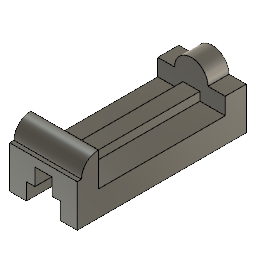
Task1 3C 2 v1 (Autodesk Fusion 360 design; units mm, degrees)
Autodesk Fusion 360 part; units mm, degrees
note: some values were not read from the file. Set by a fixed rule: which sketch regions a step uses.
sketch "Sketch1" plane through (0, 0, 0) normal (0, 0, 1) x (1, 0, 0) in component "box"
  line L0 (40, 100) -> (-40, 100)
  line L1 (-40, 100) -> (-40, -100)
  line L2 (-40, -100) -> (40, -100)
  line L3 (40, -100) -> (40, 100)
  line L4 (40, 100) -> (-40, -100) construction
  line L5 (-40, 100) -> (40, -100) construction
  dimension "d1" = 80
  dimension "d2" = 200
  constraint horizontal L0
  constraint perpendicular L0 L1
  constraint parallel L0 L2
  constraint parallel L1 L3
  constraint coincident L4 origin
  constraint coincident L5 origin
  measures "d1" distance of L1.end L2.end
  measures "d2" distance of L0.end L1.end
extrude "Extrude1" add sketch "Sketch1" along normal blind 50 in component "box"
sketch "Sketch2" plane through (0, -100, 0) normal (0, -1, 0) x (1, 0, 0) in component "box"
  line L0 (-40, 0) -> (40, 0)
  line L1 (40, 0) -> (40, 50)
  line L2 (40, 50) -> (-40, 50)
  line L3 (-40, 50) -> (-40, 0)
  line L4 (20, 0) -> (-20, 0)
  line L5 (-20, 0) -> (-20, 20)
  line L6 (-20, 20) -> (20, 20)
  line L7 (20, 20) -> (20, 0)
  line L8 (20, 0) -> (-20, 20) construction
  line L9 (-20, 0) -> (20, 20) construction
  point P0 (0, 10)
  constraint horizontal L4
  constraint perpendicular L4 L5
  constraint parallel L4 L6
  constraint parallel L5 L7
  constraint coincident L8 P0
  constraint coincident L9 P0
  constraint coincident L0 L4.start
extrude "Extrude2" cut sketch "Sketch2" against normal blind 200 contours L0 L4 L5 L6 L7 in component "box"
sketch "Sketch3" plane through (0, -100, 0) normal (0, -1, 0) x (1, 0, 0) in component "box"
  line L0 (20, 20) -> (20, 0)
  line L1 (20, 0) -> (40, 0)
  line L2 (40, 0) -> (40, 50)
  line L3 (40, 50) -> (-40, 50)
  line L4 (-40, 50) -> (-40, 0)
  line L5 (-40, 0) -> (-20, 0)
  line L6 (-20, 0) -> (-20, 20)
  line L7 (-20, 20) -> (20, 20)
  line L8 (10, 20) -> (-10, 20)
  line L9 (-10, 20) -> (-10, 40)
  line L10 (-10, 40) -> (10, 40)
  line L11 (10, 40) -> (10, 20)
  line L12 (10, 20) -> (-10, 40) construction
  line L13 (-10, 20) -> (10, 40) construction
  point P0 (0, 30)
  constraint horizontal L8
  constraint perpendicular L8 L9
  constraint parallel L8 L10
  constraint parallel L9 L11
  constraint coincident L12 P0
  constraint coincident L13 P0
  constraint coincident L7 L8.start
sketch "Sketch4" plane through (40, 0, 0) normal (1, 0, 0) x (0, 1, 0) in component "box"
  line L0 (-100, 0) -> (100, 0)
  line L1 (100, 0) -> (100, 50)
  line L2 (100, 50) -> (-100, 50)
  line L3 (-100, 50) -> (-100, 0)
  line L4 (75, 30) -> (-75, 30)
  line L5 (-75, 30) -> (-75, 50)
  line L6 (-75, 50) -> (75, 50)
  line L7 (75, 50) -> (75, 30)
  line L8 (75, 30) -> (-75, 50) construction
  line L9 (-75, 30) -> (75, 50) construction
  point P0 (0, 40)
  constraint horizontal L4
  constraint perpendicular L4 L5
  constraint parallel L4 L6
  constraint parallel L5 L7
  constraint coincident L8 P0
  constraint coincident L9 P0
extrude "Extrude3" cut sketch "Sketch4" against normal blind 80 contours L2 L4 L5 L6 L7 in component "box"
extrude "Extrude4" add sketch "Sketch3" against normal blind 200 contours L7 L8 L9 L10 L11 in component "box"
sketch "Sketch5" plane through (0, -100, 0) normal (0, -1, 0) x (1, 0, 0) in component "box"
  line L0 (-20, 20) -> (20, 20)
  line L1 (20, 20) -> (20, 0)
  line L2 (20, 0) -> (40, 0)
  line L3 (40, 0) -> (40, 50)
  line L4 (40, 50) -> (-40, 50)
  line L5 (-40, 50) -> (-40, 0)
  line L6 (-40, 0) -> (-20, 0)
  line L7 (-20, 0) -> (-20, 20)
  line L8 (10, 20) -> (-10, 20)
  line L9 (-10, 20) -> (-10, 40)
  line L10 (-10, 40) -> (10, 40)
  line L11 (10, 40) -> (10, 20)
  line L12 (10, 20) -> (-10, 40) construction
  line L13 (-10, 20) -> (10, 40) construction
  point P0 (0, 30)
  constraint horizontal L8
  constraint perpendicular L8 L9
  constraint parallel L8 L10
  constraint parallel L9 L11
  constraint coincident L12 P0
  constraint coincident L13 P0
  constraint coincident L0 L8.start
extrude "Extrude5" cut sketch "Sketch5" against normal blind 25 contours L0 L8 L9 L10 L11 in component "box"
sketch "Sketch6" plane through (0, 100, 0) normal (0, 1, 0) x (-1, 0, 0) in component "box"
  line L0 (-20, 20) -> (20, 20)
  line L1 (20, 20) -> (20, 0)
  line L2 (20, 0) -> (40, 0)
  line L3 (40, 0) -> (40, 50)
  line L4 (40, 50) -> (-40, 50)
  line L5 (-40, 50) -> (-40, 0)
  line L6 (-40, 0) -> (-20, 0)
  line L7 (-20, 0) -> (-20, 20)
  line L8 (10, 20) -> (-10, 20)
  line L9 (-10, 20) -> (-10, 40)
  line L10 (-10, 40) -> (10, 40)
  line L11 (10, 40) -> (10, 20)
  line L12 (10, 20) -> (-10, 40) construction
  line L13 (-10, 20) -> (10, 40) construction
  point P0 (0, 30)
  constraint horizontal L8
  constraint perpendicular L8 L9
  constraint parallel L8 L10
  constraint parallel L9 L11
  constraint coincident L12 P0
  constraint coincident L13 P0
  constraint coincident L0 L8.start
extrude "Extrude6" cut sketch "Sketch6" against normal blind 25 contours L0 L8 L9 L10 L11 in component "box"
sketch "Sketch7" plane through (40, 0, 0) normal (1, 0, 0) x (0, 1, 0) in component "box"
  line L0 (75, 50) -> (75, 30)
  line L1 (75, 30) -> (-75, 30)
  line L2 (-75, 30) -> (-75, 50)
  line L3 (-75, 50) -> (-100, 50)
  line L4 (-100, 50) -> (-100, 0)
  line L5 (-100, 0) -> (100, 0)
  line L6 (100, 0) -> (100, 50)
  line L7 (100, 50) -> (75, 50)
  circle A0 centre (-75, 50) radius 20
  constraint coincident L2.end L3.start
extrude "Extrude7" add sketch "Sketch7" against normal blind 80 contours L2 L3 A0 picked at (-86.5147, 56.648) in component "box"
sketch "Sketch8" plane through (0, 100, 0) normal (0, 1, 0) x (-1, 0, 0) in component "box"
  line L0 (10, 40) -> (10, 20)
  line L1 (10, 20) -> (20, 20)
  line L2 (20, 20) -> (20, 0)
  line L3 (20, 0) -> (40, 0)
  line L4 (40, 0) -> (40, 50)
  line L5 (40, 50) -> (-40, 50)
  line L6 (-40, 50) -> (-40, 0)
  line L7 (-40, 0) -> (-20, 0)
  line L8 (-20, 0) -> (-20, 20)
  line L9 (-20, 20) -> (-10, 20)
  line L10 (-10, 20) -> (-10, 40)
  line L11 (-10, 40) -> (10, 40)
  circle A0 centre (0.1969, 50) radius 19.8031
  constraint coincident L5 A0.centre
extrude "Extrude8" add sketch "Sketch8" against normal blind 25 contours L5 A0 in component "box"
sketch "Sketch9" plane through (40, 0, 0) normal (1, 0, 0) x (0, 1, 0) in component "box"
  line L0 (75, 50) -> (75, 30)
  line L1 (75, 30) -> (-75, 30)
  arc A0 (-75, 30) -> (-95, 50) centre (-75, 50) ccw
  line L2 (-95, 50) -> (-100, 50)
  line L3 (-100, 50) -> (-100, 0)
  line L4 (-100, 0) -> (100, 0)
  line L5 (100, 0) -> (100, 50)
  line L6 (100, 50) -> (75, 50)
  line L7 (75, 30) -> (-75, 30)
  line L8 (-75, 30) -> (-75, 70)
  line L9 (-75, 70) -> (75, 70)
  line L10 (75, 70) -> (75, 30)
  line L11 (75, 30) -> (-75, 70) construction
  line L12 (-75, 30) -> (75, 70) construction
  point P0 (0, 50)
  constraint horizontal L7
  constraint perpendicular L7 L8
  constraint parallel L7 L9
  constraint parallel L8 L10
  constraint coincident L11 P0
  constraint coincident L12 P0
  constraint coincident L0.end L1.start
extrude "Extrude9" cut sketch "Sketch9" against normal blind 80 contours A0 L8 in component "box"
sketch "Sketch10" plane through (0, -100, 0) normal (0, -1, 0) x (1, 0, 0) in component "box"
  line L0 (10, 40) -> (10, 20)
  line L1 (10, 20) -> (20, 20)
  line L2 (20, 20) -> (20, 0)
  line L3 (20, 0) -> (40, 0)
  line L4 (40, 0) -> (40, 50)
  line L5 (40, 50) -> (-40, 50)
  line L6 (-40, 50) -> (-40, 0)
  line L7 (-40, 0) -> (-20, 0)
  line L8 (-20, 0) -> (-20, 20)
  line L9 (-20, 20) -> (-10, 20)
  line L10 (-10, 20) -> (-10, 40)
  line L11 (-10, 40) -> (10, 40)
  line L12 (10, 20) -> (-10, 20)
  line L13 (-10, 20) -> (-10, 40)
  line L14 (-10, 40) -> (10, 40)
  line L15 (10, 40) -> (10, 20)
  line L16 (10, 20) -> (-10, 40) construction
  line L17 (-10, 20) -> (10, 40) construction
  point P0 (0, 30)
  constraint horizontal L12
  constraint perpendicular L12 L13
  constraint parallel L12 L14
  constraint parallel L13 L15
  constraint coincident L16 P0
  constraint coincident L17 P0
  constraint coincident L0.end L1.start
extrude "Extrude10" add sketch "Sketch10" against normal blind 50 contours L0 L10 L11 L12 L13 L14 L15 in component "box"
sketch "Sketch11" plane through (0, -100, 0) normal (0, -1, 0) x (1, 0, 0) in component "box"
  line L0 (-20, 20) -> (20, 20)
  line L1 (20, 20) -> (20, 0)
  line L2 (20, 0) -> (40, 0)
  line L3 (40, 0) -> (40, 50)
  line L4 (40, 50) -> (-40, 50)
  line L5 (-40, 50) -> (-40, 0)
  line L6 (-40, 0) -> (-20, 0)
  line L7 (-20, 0) -> (-20, 20)
  line L8 (10, 20) -> (-10, 20)
  line L9 (-10, 20) -> (-10, 40)
  line L10 (-10, 40) -> (10, 40)
  line L11 (10, 40) -> (10, 20)
  line L12 (10, 20) -> (-10, 40) construction
  line L13 (-10, 20) -> (10, 40) construction
  point P0 (0, 30)
  constraint horizontal L8
  constraint perpendicular L8 L9
  constraint parallel L8 L10
  constraint parallel L9 L11
  constraint coincident L12 P0
  constraint coincident L13 P0
  constraint coincident L0 L8.start
extrude "Extrude11" cut sketch "Sketch11" against normal blind 25 contours L0 L8 L9 L10 L11 in component "box"
component "box" placed x (1, 0, 0) y (0, 1, 0) z (0, 0, 1) at (0, 0, 0)
